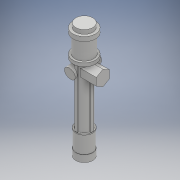
# Autodesk Inventor part: らっくあんどぴにおん
Saved by Autodesk Inventor 2018 (Build 220112000, 112)
## iProperties
Created: 2017-09-09
Part Number: らっくあんどぴにおん
Material: 一般
Document SubType Name: Modeling
Designer: Kenta
Density: 1 g/cm^3
Appearance: 既定
Author: Kenta
Autodesk Inventor part; units mm, degrees
ref_plane "YZ Plane" through (0, 0, 0) normal (1, 0, 0) x (0, 1, 0)
ref_plane "XZ Plane" through (0, 0, 0) normal (0, 1, 0) x (-1, 0, 0)
ref_plane "XY Plane" through (0, 0, 0) normal (0, 0, 1) x (1, 0, 0)
sketch "スケッチ5" plane through (0, 0, 0) normal (0, 0, 1) x (1, 0, 0)
  circle A0 centre (0, 0) radius 25
  dimension "d14" = 50
  constraints: 1 centre point, 1 coincident
  measures "d14" diameter of A0
extrude "押し出し4" add sketch "スケッチ5" along normal blind 20
sketch "スケッチ6" plane through (0, 0, 20) normal (0, 0, 1) x (1, 0, 0)
  circle A0 centre (0, 0) radius 24
  dimension "d17" = 48
  constraints: 1 centre point, 1 coincident
  measures "d17" diameter of A0
extrude "押し出し5" add sketch "スケッチ6" along normal blind 50
sketch "スケッチ7" plane through (0, 0, 70) normal (0, 0, 1) x (1, 0, 0)
  circle A0 centre (0, 0) radius 25
  dimension "d20" = 50
  constraints: 1 centre point, 1 coincident
  measures "d20" diameter of A0
extrude "押し出し6" add sketch "スケッチ7" along normal blind 3
sketch "スケッチ8" plane through (0, 0, 73) normal (0, 0, 1) x (1, 0, 0)
  line L0 (4.5, 23.5744) -> (4.5, 20.5122)
  line L1 (-4.5, 20.5122) -> (-4.5, 23.5744)
  line L2 (-4.5, 23.7345) -> (-4.2984, 23.6119) construction
  line L3 (4.5, 23.7345) -> (4.2984, 23.6119) construction
  line L4 (20.5122, 4.5) -> (23.5744, 4.5)
  line L5 (23.5744, -4.5) -> (20.5122, -4.5)
  line L6 (-23.5744, 4.5) -> (-20.5122, 4.5)
  line L7 (-20.5122, -4.5) -> (-23.5744, -4.5)
  line L8 (4.5, -20.5122) -> (4.5, -23.5744)
  line L9 (-4.5, -23.5744) -> (-4.5, -20.5122)
  arc A0 (23.5744, -4.5) -> (23.5744, 4.5) centre (0, 0) ccw
  arc A1 (4.5, 23.5744) -> (-4.5, 23.5744) centre (0, 0) ccw
  arc A2 (-23.5744, 4.5) -> (-23.5744, -4.5) centre (0, 0) ccw
  arc A3 (-4.5, -23.5744) -> (4.5, -23.5744) centre (0, 0) ccw
  arc A4 (-20.5122, -4.5) -> (-4.5, -20.5122) centre (0, 0) ccw
  arc A5 (4.5, -20.5122) -> (20.5122, -4.5) centre (0, 0) ccw
  arc A6 (20.5122, 4.5) -> (4.5, 20.5122) centre (0, 0) ccw
  arc A7 (-4.5, 20.5122) -> (-20.5122, 4.5) centre (0, 0) ccw
  constraints: 21 end point, 18 point on circle, 8 centre point, 4 parallel, 2 coincident, 2 horizontal
extrude "押し出し7" add sketch "スケッチ8" along normal blind 130
sketch "スケッチ11" plane through (0, 0, 0) normal (1, 0, 0) x (0, 1, 0)
  line L0 (4.5, 203) -> (-4.5, 203) projected
  line L1 (0, 203) -> (-19.4856, 214.25)
  line L2 (-19.4856, 214.25) -> (-19.4856, 236.75)
  line L3 (-19.4856, 236.75) -> (0, 248)
  line L4 (0, 248) -> (19.4856, 236.75)
  line L5 (19.4856, 236.75) -> (19.4856, 214.25)
  line L6 (19.4856, 214.25) -> (0, 203)
  point P0 (0, 0)
  point P1 (0, 225.5)
  point P2 (0, 225.5)
  dimension "d66" = 19.4856
  constraints: 12 end point, 1 coincident, 1 midpoint, 13 other
  measures "d66" distance from line of L2 point (0, 225.5)
extrude "押し出し8" add sketch "スケッチ11" along normal blind 55
ref_plane "作業平面4" through (0, 0, 260) normal (0, 0, 1) x (1, 0, 0)
sketch "スケッチ12" plane through (0, 0, 260) normal (0, 0, 1) x (1, 0, 0)
  circle A0 centre (0, 0) radius 27
  dimension "d36" = 54
  constraints: 1 centre point, 1 coincident
  measures "d36" diameter of A0
extrude "押し出し9" add sketch "スケッチ12" along normal blind 54
sketch "スケッチ13" plane through (0, 0, 260) normal (0, 0, 1) x (1, 0, 0)
  line L0 (0, 0) -> (0, -19.4856) projected
  circle A0 centre (0, 0) radius 33
  dimension "d39" = 66
  constraints: 1 centre point, 1 coincident
  measures "d39" diameter of A0
extrude "押し出し10" add sketch "スケッチ13" against normal blind 10
sketch "スケッチ14" plane through (0, 0, 314) normal (0, 0, 1) x (1, 0, 0)
  line L0 (0, -19.4856) -> (0, 0) projected
  circle A0 centre (0, 0) radius 33
  dimension "d42" = 66
  constraints: 1 centre point, 1 coincident
  measures "d42" diameter of A0
extrude "押し出し11" add sketch "スケッチ14" along normal blind 13
sketch "スケッチ15" plane through (0, 0, 327) normal (0, 0, 1) x (1, 0, 0)
  circle A0 centre (0, 0) radius 25
  dimension "d45" = 50
  constraints: 1 centre point, 1 coincident
  measures "d45" diameter of A0
extrude "押し出し12" add sketch "スケッチ15" along normal blind 12
ref_plane "作業平面6" through (0, 44.2483, 217.6861) normal (0, 0.9905095, 0.1374445) x (1, 0, 0)
ref_plane "作業平面5" through (0, 19.4856, 214.25) normal (0, 0.9905095, 0.1374445) x (1, 0, 0)
sketch "スケッチ16" plane through (0, 44.2483, 217.6861) normal (0, 0.9905095, 0.1374445) x (1, 0, 0)
  circle A0 centre (-13, -10.0889) radius 21
  point P0 (0, 209.5385)
  point P1 (0, -38.0889)
  dimension "d50" = 28
  dimension "d51" = 42
  constraints: 1 centre point, 1 coincident
  measures "d50" vertical distance of point (0, -38.089) point (-13, -10.089)
  measures "d51" diameter of A0
extrude "押し出し13" add sketch "スケッチ16" against normal blind 27
sketch "スケッチ17" plane through (-13, 42.8616, 227.6793) normal (0, 0.9905095, 0.1374445) x (1, 0, 0)
  circle A0 centre (0, 0) radius 16
  point P0 (13, 219.6274)
  dimension "d54" = 32
  constraints: 1 centre point
  measures "d54" diameter of A0
extrude "押し出し14" add sketch "スケッチ17" against normal blind 73
sketch "スケッチ18" plane through (-13, 42.8616, 227.6793) normal (0, 0.9905095, 0.1374445) x (1, 0, 0)
  point P0 (13, 219.6274)
  point P1 (0, 0)
hole "穴1" at (-13, 42.8616, 227.6793) direction (0, -0.9905095, -0.1374445) diameter 15 depth 70
sketch "スケッチ19" plane through (0, 0, 203) normal (0, 0, 1) x (1, 0, 0)
  line L0 (4.5, 23.5744) -> (4.5, 20.5122)
  line L1 (-4.5, 20.5122) -> (-4.5, 23.5744)
  line L2 (-4.5, 23.7345) -> (-4.2984, 23.6119) construction
  line L3 (4.5, 23.7345) -> (4.2984, 23.6119) construction
  line L4 (20.5122, 4.5) -> (23.5744, 4.5)
  line L5 (23.5744, -4.5) -> (20.5122, -4.5)
  line L6 (-23.5744, 4.5) -> (-20.5122, 4.5)
  line L7 (-20.5122, -4.5) -> (-23.5744, -4.5)
  line L8 (4.5, -20.5122) -> (4.5, -23.5744)
  line L9 (-4.5, -23.5744) -> (-4.5, -20.5122)
  arc A0 (23.5744, -4.5) -> (23.5744, 4.5) centre (0, 0) ccw
  arc A1 (4.5, 23.5744) -> (-4.5, 23.5744) centre (0, 0) ccw
  arc A2 (-23.5744, 4.5) -> (-23.5744, -4.5) centre (0, 0) ccw
  arc A3 (-4.5, -23.5744) -> (4.5, -23.5744) centre (0, 0) ccw
  arc A4 (-20.5122, -4.5) -> (-4.5, -20.5122) centre (0, 0) ccw
  arc A5 (4.5, -20.5122) -> (20.5122, -4.5) centre (0, 0) ccw
  arc A6 (20.5122, 4.5) -> (4.5, 20.5122) centre (0, 0) ccw
  arc A7 (-4.5, 20.5122) -> (-20.5122, 4.5) centre (0, 0) ccw
  line L10 (4.5, 23.5744) -> (4.5, 20.5122)
  line L11 (-4.5, 20.5122) -> (-4.5, 23.5744)
  line L12 (-4.5, 23.7345) -> (-4.2984, 23.6119) construction
  line L13 (4.5, 23.7345) -> (4.2984, 23.6119) construction
  line L14 (20.5122, 4.5) -> (23.5744, 4.5)
  line L15 (23.5744, -4.5) -> (20.5122, -4.5)
  line L16 (-23.5744, 4.5) -> (-20.5122, 4.5)
  line L17 (-20.5122, -4.5) -> (-23.5744, -4.5)
  line L18 (4.5, -20.5122) -> (4.5, -23.5744)
  line L19 (-4.5, -23.5744) -> (-4.5, -20.5122)
  arc A8 (23.5744, -4.5) -> (23.5744, 4.5) centre (0, 0) ccw
  arc A9 (4.5, 23.5744) -> (-4.5, 23.5744) centre (0, 0) ccw
  arc A10 (-23.5744, 4.5) -> (-23.5744, -4.5) centre (0, 0) ccw
  arc A11 (-4.5, -23.5744) -> (4.5, -23.5744) centre (0, 0) ccw
  arc A12 (-20.5122, -4.5) -> (-4.5, -20.5122) centre (0, 0) ccw
  arc A13 (4.5, -20.5122) -> (20.5122, -4.5) centre (0, 0) ccw
  arc A14 (20.5122, 4.5) -> (4.5, 20.5122) centre (0, 0) ccw
  arc A15 (-4.5, 20.5122) -> (-20.5122, 4.5) centre (0, 0) ccw
  constraints: 42 end point, 36 point on circle, 16 centre point, 8 parallel, 4 coincident, 4 horizontal
extrude "押し出し15" add sketch "スケッチ19" along normal blind 47
